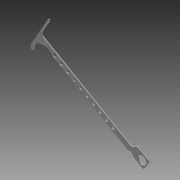
# Autodesk Inventor part: passive hooks arpan style.iam
Saved by Autodesk Inventor 2013 (Build 170138000, 138)
## iProperties
Created: 2013-02-09
Part Number: passive hooks arpan style.iam
Material: Steel
Document SubType Name: Modeling
Designer: Arpan
Density: 7.85 g/cm^3
Mass: 379.399 g
Surface Area: 263.535 cm^2
Volume: 48.3311 cm^3
Author: Arpan
Autodesk Inventor part; units mm, degrees
ref_plane "YZ Plane" through (0, 0, 0) normal (1, 0, 0) x (0, 1, 0)
ref_plane "XZ Plane" through (0, 0, 0) normal (0, 1, 0) x (-1, 0, 0)
ref_plane "XY Plane" through (0, 0, 0) normal (0, 0, 1) x (1, 0, 0)
sketch "Sketch1" plane through (0, 0, 0) normal (0, 0, 1) x (1, 0, 0)
  line L0 (0, 0) -> (-65.4914, 0)
  line L1 (-35.9207, 0) -> (-35.9207, 19.05)
  arc A0 (0, 0) -> (-71.8414, 0) centre (-35.9207, -24.341) ccw
  line L2 (0, 0) -> (307.9586, -177.8)
  line L3 (0, 0) -> (60.0796, 0)
  line L4 (0, 0) -> (293.1106, -169.2275)
  line L5 (293.1106, -169.2275) -> (302.6356, -152.7297)
  circle A1 centre (302.6356, -152.7297) radius 14.2875
  line L6 (307.9586, -177.8) -> (327.0086, -144.8044)
  line L7 (327.0086, -144.8044) -> (283.0145, -119.4044)
  line L8 (283.0145, -119.4044) -> (273.4895, -135.9022)
  line L9 (273.4895, -135.9022) -> (-4.8088, 24.7734)
  line L10 (-4.8088, 24.7734) -> (-21.3066, 34.2984)
  line L11 (-21.3066, 34.2984) -> (-37.8044, 43.8234)
  line L12 (-37.8044, 43.8234) -> (-48.8029, 50.1734)
  line L13 (-77.7706, 0) -> (-48.8029, 50.1734)
  line L14 (-71.8414, -12.7) -> (-77.7706, -12.7)
  line L15 (-77.7706, -12.7) -> (-77.7706, 0)
  line L16 (-65.4914, 0) -> (-65.4914, -12.7)
  line L17 (-65.4914, -12.7) -> (-71.8414, -12.7)
  line L18 (-65.4914, 0) -> (-65.4914, 7.4136)
  dimension "d0" = 71.8414
  dimension "d1" = 19.05
  dimension "d3" = 30
  dimension "d4" = 355.6
  dimension "d5" = 338.455
  dimension "d6" = 19.05
  dimension "d7" = 28.575
  dimension "d9" = 38.1
  dimension "d10" = 50.8
  dimension "d11" = 19.05
  dimension "d12" = 19.05
  dimension "d13" = 19.05
  dimension "d14" = 12.7
  dimension "d17" = 12.7
  dimension "d31" = 6.35
  constraints: 38 end point, 6 perpendicular, 4 point on circle, 3 collinear, 3 parallel, 2 centre point, 2 point on line, 1 coincident, 1 horizontal
  measures "d0" distance of L0.start A0.end
  measures "d1" distance of L1.start L1.end
  measures "d3" angle of L2 L3
  measures "d4" distance of L0.start L2.end
  measures "d5" distance of L0.start L4.end
  measures "d6" distance of L4.end L5.end
  measures "d7" diameter of A1
  measures "d9" distance of L2.end L6.end
  measures "d10" distance of L6.end L7.end
  measures "d11" distance of L7.end L8.end
  measures "d12" distance of L9.end L10.end
  measures "d13" distance of L10.end L11.end
  measures "d14" distance of L11.end L12.end
  measures "d17" distance of A0.end L14.start
  measures "d31" distance of L0.end A0.end
extrude "Extrusion1" add sketch "Sketch1" along normal blind 3.175 contours L3 L9 L8 L7 L6 L2 | A0 L18 L16 L17 L14 L15 L13 L12 L11 L10 L9 L3
fillet "Fillet1" radius 3.175 1 edges at (-77.7706, 0, 1.5875)
sketch "Sketch2" plane through (0, 0, 3.175) normal (0, 0, 1) x (1, 0, 0)
  line L0 (-48.8029, 50.1734) -> (-77.3452, 0.7368) projected
  line L1 (273.4895, -135.9022) -> (268.727, -144.1511)
  circle A0 centre (268.727, -144.1511) radius 6.35
  line L2 (268.727, -144.1511) -> (261.5833, -140.0267)
  circle A1 centre (246.73, -131.4511) radius 6.35
  circle A2 centre (224.733, -118.7511) radius 6.35
  circle A3 centre (202.7359, -106.0511) radius 6.35
  circle A4 centre (180.7389, -93.3511) radius 6.35
  circle A5 centre (158.7418, -80.6511) radius 6.35
  circle A6 centre (136.7448, -67.9511) radius 6.35
  circle A7 centre (114.7477, -55.2511) radius 6.35
  circle A8 centre (92.7507, -42.5511) radius 6.35
  circle A9 centre (70.7536, -29.8511) radius 6.35
  circle A10 centre (48.7566, -17.1511) radius 6.35
  circle A11 centre (26.7595, -4.4511) radius 6.35
  circle A12 centre (4.7625, 8.2489) radius 6.35
  dimension "d19" = 9.525
  dimension "d20" = 12.7
  dimension "d23" = 25.4
  constraints: 13 centre point, 4 end point, 1 coincident, 1 parallel, 1 perpendicular, 25 other
  measures "d19" distance of L1.start L1.end
  measures "d20" diameter of A0
  measures "d23" distance of L2.start A1.centre
extrude "Extrusion2" cut sketch "Sketch2" against normal blind 25.4
fillet "Fillet2" radius 6.35 3 edges at (283.0145, -119.4044, 1.5875) (327.0086, -144.8044, 1.5875) (307.9586, -177.8, 1.5875)
fillet "Fillet3" radius 12.7 1 edges at (-65.4914, 7.4136, 1.5875)
sketch "Sketch7" plane through (0, 0, 3.175) normal (0, 0, 1) x (1, 0, 0)
  line L0 (273.4895, -135.9022) -> (-48.8029, 50.1734) projected
  line L1 (-48.8029, 50.1734) -> (-18.0523, 105.731)
  line L2 (-18.0523, 105.731) -> (-12.4965, 102.656)
  line L3 (-12.4965, 102.656) -> (-44.2988, 47.5729)
  dimension "d42" = 63.5
  dimension "d43" = 6.35
  constraints: 6 end point, 2 perpendicular, 1 point on line
  measures "d42" distance of L0.end L1.end
  measures "d43" distance of L1.end L2.end
extrude "Extrusion5" add sketch "Sketch7" against normal blind 3.175
sketch "Sketch8" plane through (0, 0, 3.175) normal (0, 0, 1) x (1, 0, 0)
  line L0 (273.4895, -135.9022) -> (-44.2988, 47.5729) projected
  line L1 (-48.8029, 50.1734) -> (-77.3452, 0.7368) projected
  line L2 (-48.8029, 50.1734) -> (-51.9779, 44.6742)
  line L3 (-51.9779, 44.6742) -> (-27.2313, 30.3867)
  circle A0 centre (-27.2313, 30.3867) radius 3.175
  dimension "d46" = 6.35
  dimension "d47" = 28.575
  dimension "d48" = 6.35
  constraints: 4 end point, 1 centre point, 1 coincident, 1 parallel, 1 point on line
  measures "d46" distance of L1.start L2.end
  measures "d47" distance of L2.end L3.end
  measures "d48" diameter of A0
extrude "Extrusion6" cut sketch "Sketch8" against normal blind 6.35
fillet "Fillet4" radius 12.7 1 edges at (-44.2988, 47.5729, 1.5875)
fillet "Fillet5" radius 3.175 2 edges at (-12.4965, 102.656, 1.5875) (-18.0523, 105.731, 1.5875)
sketch "Sketch9" plane through (0, 0, 3.175) normal (0, 0, 1) x (1, 0, 0)
  circle A0 centre (246.73, -131.4511) radius 6.35 projected
  circle A1 centre (268.727, -144.1511) radius 6.35 projected
  circle A2 centre (224.733, -118.7511) radius 6.35 projected
extrude "Extrusion7" add sketch "Sketch9" against normal blind 3.175
sketch "Sketch10" plane through (0, 0, 3.175) normal (0, 0, 1) x (1, 0, 0)
  line L0 (0, 0) -> (302.4594, -174.625) projected
  line L1 (264.1907, -173.1439) -> (264.634, -147.7477) projected
  line L2 (264.634, -147.7477) -> (239.2379, -147.3044) projected
  line L3 (251.9359, -147.5261) -> (264.5469, -152.7362)
  constraints: 2 end point, 2 point on line, 1 midpoint
extrude "Extrusion8" cut sketch "Sketch10" against normal blind 6.35
fillet "Fillet6" radius 3.175 1 edges at (264.5469, -152.7362, 1.5875)
sketch "Sketch11" plane through (0, 0, 3.175) normal (0, 0, 1) x (1, 0, 0)
  arc A0 (264.5796, -150.8663) -> (266.1666, -153.6713) centre (267.7541, -150.9217) ccw projected
  line L0 (266.1666, -153.6713) -> (302.4594, -174.625) projected
  line L1 (264.634, -147.7477) -> (264.5796, -150.8663) projected
  line L2 (264.634, -147.7477) -> (267.8085, -147.8031)
  line L3 (267.8085, -147.8031) -> (267.6907, -154.5513)
  dimension "d58" = 3.175
  constraints: 4 end point, 2 perpendicular, 1 point on line
  measures "d58" distance of L1.start L2.end
extrude "Extrusion9" cut sketch "Sketch11" against normal blind 6.35
fillet "Fillet7" radius 19.05 1 edges at (273.4895, -135.9022, 1.5875)
fillet "Fillet8" radius 19.05 1 edges at (255.6345, -147.5907, 1.5875)
fillet "Fillet9" radius 19.05 1 edges at (267.6907, -154.5513, 1.5875)
fillet "Fillet10" radius 3.175 1 edges at (267.8085, -147.8031, 1.5875)
sketch "Sketch12" plane through (0, 0, 3.175) normal (0, 0, 1) x (1, 0, 0)
  arc A0 (0, 0) -> (-59.7725, 11.9064) centre (-35.9207, -24.341) ccw projected
  arc A1 (0, 0) -> (-35.9207, 19.05) centre (-32.7383, -18.3402) ccw
  constraints: 3 point on circle, 1 centre point
extrude "Extrusion10" cut sketch "Sketch12" against normal blind 6.35
body "Solid1"
